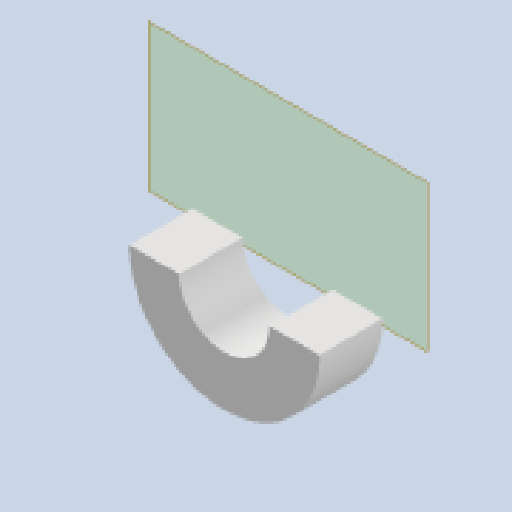
# Autodesk Inventor part: верх штуки для подшипников
Saved by Autodesk Inventor 2024.2 (Build 282272000, 272)
## iProperties
Created: 2025-11-24
Part Number: верх штуки для подшипников
Material: Типовые
Document SubType Name: Modeling
Designer: katya_notebook
Density: 1 g/cm^3
Appearance: По умолчанию
Author: katya_notebook
Autodesk Inventor part; units mm, degrees
ref_plane "YZ Plane" through (0, 0, 0) normal (1, 0, 0) x (0, 1, 0)
ref_plane "XZ Plane" through (0, 0, 0) normal (0, 1, 0) x (-1, 0, 0)
ref_plane "XY Plane" through (0, 0, 0) normal (0, 0, 1) x (1, 0, 0)
ref_plane "РабПлоскость1" through (-89.0227, 116.8233, -154.317) normal (0, 0, -1) x (-1, 0, 0)
sketch "Эскиз1" plane through (-89.0227, 116.8233, -154.317) normal (0, 0, -1) x (-1, 0, 0)
  arc A0 (7.1, -10.5) -> (-7.1, -10.5) centre (0, -10.5) ccw projected
  line L0 (7.1, -10.5) -> (15, -10.5) projected
  line L1 (15, -10.5) -> (15, 7.5) projected
  line L2 (15, 7.5) -> (20, 7.5) projected
  line L3 (20, 7.5) -> (20, 10.5) projected
  line L4 (20, 10.5) -> (-20, 10.5) projected
  line L5 (-20, 10.5) -> (-20, 7.5) projected
  line L6 (-20, 7.5) -> (-15, 7.5) projected
  line L7 (-15, 7.5) -> (-15, -10.5) projected
  line L8 (-15, -10.5) -> (-7.1, -10.5) projected
  circle A1 centre (0, -10.5) radius 15
  line L9 (15, -10.5) -> (-15, -10.5)
  circle A2 centre (0, -10.5) radius 7 projected
  circle A3 centre (0, -10.5) radius 7.1
  line L10 (15, -10.5) -> (-15, -10.5)
  point P0 (-89.0227, -116.8233)
  point P1 (-7.1, -10.5)
  constraints: 4 end point, 2 coincident, 2 point on circle, 1 centre point, 1 horizontal, 3 other
extrude "Выдавливание1" add sketch "Эскиз1" against normal blind 10 contours L0 A1 L8 A3
ref_plane "РабПлоскость2" through (-89.2672, 127.3233, -149.317) normal (0, -1, 0) x (1, 0, 0)
sketch "Эскиз2" plane through (-89.2672, 127.3233, -149.317) normal (0, -1, 0) x (1, 0, 0)
  circle A0 centre (11.2445, 0) radius 2
  line L0 (-14.7555, -5) -> (15.2445, -5) projected
  line L1 (15.2445, -5) -> (15.2445, 5) projected
  line L2 (-6.8555, 5) -> (7.3445, 5) projected
  line L3 (-0.0139, 5) -> (-0.0139, -5)
  circle A1 centre (-11.2723, 0) radius 2
  point P0 (89.2672, 149.317)
  dimension "d2" = 4
  dimension "d3" = 5
  dimension "d4" = 4
  constraints: 2 centre point, 2 end point, 2 point on line, 1 perpendicular, 1 symmetric about line, 1 other
  measures "d2" diameter of A0
  measures "d3" distance from line of L0 A0.centre
  measures "d4" distance from line of L1 A0.centre
extrude "Выдавливание2" cut sketch "Эскиз2" along normal blind 51.5
